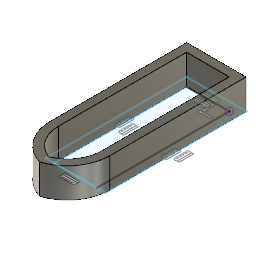
boat v2 (Autodesk Fusion 360 design; units mm, degrees)
Autodesk Fusion 360 part; units mm, degrees
note: some values were not read from the file. Chosen so that the rebuilt part matches the saved one: which face or edge a step refers to.
sketch "Sketch1" plane through (0, 0, 0) normal (0, 0, 1) x (1, 0, 0)
  line L0 (0, 0) -> (-10, 0)
  line L1 (-10, 0) -> (-10, -30)
  line L2 (-10, -30) -> (0, -30)
  line L3 (0, -30) -> (0, 0)
  arc A0 (-5, -37.3493) -> (0, -30) centre (-7.9012, -30) ccw
  arc A1 (-10, -30) -> (-5, -37.3493) centre (-2.0988, -30) ccw
  line L4 (2, -30) -> (2, 2)
  line L5 (2, 2) -> (-12, 2)
  line L6 (-12, 2) -> (-12, -30)
  arc A2 (-12, -30) -> (-5, -39.4666) centre (-2.0988, -30) ccw
  arc A3 (-5, -39.4666) -> (2, -30) centre (-7.9012, -30) ccw
  dimension "d1" = 30
  dimension "d2" = 10
  dimension "d3" = 2
  dimension "d4" = 2
  dimension "d24" = 7.3493
  dimension "d25" = 7.9012
  constraint horizontal L0
  constraint vertical L1
  constraint horizontal L2
  constraint vertical L3
  constraint coincident L0.start L3.end
  constraint tangent L3 A0
  constraint tangent L1 A1
  measures "d1" distance of L0.start L2.end
  measures "d2" distance of L0.start L0.end
  measures "d24" distance of L2 A0.start
  measures "d25" radius of A1
extrude "Extrude1" add sketch "Sketch1" along normal blind 7
sketch "Sketch2" plane through (0, 0, 0) normal (0, 0, 1) x (1, 0, 0)
  line L0 (0, 0) -> (-10, 0)
  line L1 (-10, 0) -> (-10, -31)
  line L2 (-10, -31) -> (0, -31)
  line L3 (0, -31) -> (0, 0)
  line L4 (-12, 2) -> (2, 2)
  line L5 (2, 2) -> (2, -31)
  line L6 (2, -31) -> (-12, -31)
  line L7 (-12, -31) -> (-12, 2)
  constraint horizontal L0
  constraint vertical L1
  constraint horizontal L2
  constraint vertical L3
  constraint coincident L0.start L3.end
  constraint horizontal L4
  constraint vertical L5
  constraint horizontal L6
  constraint vertical L7
extrude "Extrude2" [rolled back] along distance -3 taper angle 0
sketch "Sketch3" plane through (0, 0, 0) normal (0, 0, 1) x (1, 0, 0)
  line L0 (-5, -31) -> (2, -31)
  line L1 (2, -31) -> (-12, -31)
  line L2 (-12, -31) -> (-5, -39.5)
  line L3 (2, -31) -> (-5, -39.5)
extrude "Extrude3" [rolled back] along distance -3 taper angle 0
fillet "Fillet1" [rolled back] radius 2.5
sketch "Sketch4" plane through (0, 0, 0) normal (0, 0, 1) x (1, 0, 0)
  line L0 (-6, -14) -> (-4, -14)
  line L1 (-4, -14) -> (-4, -16)
  line L2 (-4, -16) -> (-6, -16)
  line L3 (-6, -16) -> (-6, -14)
  constraint horizontal L0
  constraint vertical L1
  constraint horizontal L2
  constraint vertical L3
extrude "Extrude4" [rolled back] along distance 40 taper angle 0
sketch "Sketch5" plane through (0, 0, 0) normal (1, 0, 0) x (0, 1, 0)
  line L0 (-16, 15) -> (-30, 15)
  line L1 (-30, 15) -> (-16, 40)
  line L2 (-16, 40) -> (-16, 15)
  constraint horizontal L0
  constraint perpendicular L0 L2
extrude "Extrude5" [rolled back] along distance -6 taper angle 0
move_face "OffsetFaces1" [rolled back] distance -4
sketch "Sketch6" plane through (0, 0, 0) normal (1, 0, 0) x (0, 1, 0)
  line L0 (-16, 41) -> (-35, 41)
  line L1 (-35, 41) -> (-35, 16)
  line L2 (-35, 16) -> (-14, 16)
  line L3 (-16, 41) -> (-16, 16)
  constraint horizontal L0
  constraint perpendicular L0 L1
  constraint perpendicular L1 L2
  constraint coincident L2 L3.end
  constraint perpendicular L2 L3
extrude "Extrude6" [rolled back] along distance -23 taper angle 0
sketch "Sketch7" plane through (-6, 0, 0) normal (-1, 0, 0) x (0, -1, 0)
  line L0 (29.44, 16) -> (16, 16)
  line L1 (16, 16) -> (16, 40)
  line L2 (16, 40) -> (14, 40)
  line L3 (14, 40) -> (14, 0)
  line L4 (14, 0) -> (16, 0)
  line L5 (16, 0) -> (16, 15)
  line L6 (16, 15) -> (30, 15)
  line L7 (30, 15) -> (29.44, 16)
  line L8 (16, 40) -> (30, 34)
  line L9 (30, 34) -> (35, 24)
  line L10 (35, 24) -> (35, 18)
  line L11 (35, 18) -> (33.2438, 13.9022)
  line L12 (33.2438, 13.9022) -> (16, 13.9022)
  constraint coincident L1.end L2.start
  constraint perpendicular L2 L10
  constraint perpendicular L8 L11
  constraint coincident L1 L12.end
  constraint perpendicular L1 L12
extrude "Extrude7" [rolled back] along distance -2 taper angle 0
sketch "Sketch8" plane through (-6, 0, 0) normal (-1, 0, 0) x (0, -1, 0)
  line L0 (16, 13.9022) -> (33.2438, 13.9022)
  line L1 (33.2438, 13.9022) -> (35, 18)
  line L2 (35, 18) -> (35, 24)
  line L3 (35, 24) -> (30, 34)
  line L4 (30, 34) -> (16, 40)
  line L5 (16, 40) -> (14, 40)
  line L6 (14, 40) -> (14, 0)
  line L7 (14, 0) -> (16, 0)
  line L8 (16, 0) -> (16, 13.9022)
  line L9 (16, 40) -> (33.2438, 13.9022)
  constraint coincident L4.end L5.start
  constraint coincident L0.end L1.start
extrude "Extrude8" [rolled back] along distance -2 taper angle 0
